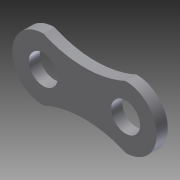
# Autodesk Inventor part: outter_link
Saved by Autodesk Inventor 2011 SP1 (Build 150282100, 282)
## iProperties
Created: 2013-01-14
Part Number: outter_link
Document SubType Name: Modeling
Designer: 971065
Density: 1 g/cm^3
Author: 971065
Autodesk Inventor part; units mm, degrees
ref_plane "YZ Plane" through (0, 0, 0) normal (1, 0, 0) x (0, 1, 0)
ref_plane "XZ Plane" through (0, 0, 0) normal (0, 1, 0) x (-1, 0, 0)
ref_plane "XY Plane" through (0, 0, 0) normal (0, 0, 1) x (1, 0, 0)
sketch "Sketch1" plane through (0, 0, 0) normal (0, 0, 1) x (1, 0, 0)
  arc A0 (-14.097, 3.556) -> (-14.097, -3.556) centre (-14.097, 0) ccw
  arc A1 (-4.699, -3.556) -> (-4.699, 3.556) centre (-4.699, 0) ccw
  line L0 (-9.398, -2.54) -> (-9.398, 2.54)
  arc A2 (-14.097, 3.556) -> (-4.699, 3.556) centre (-9.398, 13.9144) ccw
  arc A3 (-4.699, -3.556) -> (-14.097, -3.556) centre (-9.398, -13.9144) ccw
  circle A4 centre (-14.097, 0) radius 1.651
  circle A5 centre (-4.699, 0) radius 1.651
  point P0 (0, 0)
  dimension "d0" = 7.112
  dimension "d1" = 7.112
  dimension "d5" = 9.398
  dimension "d6" = 4.699
  dimension "d8" = 5.08
  dimension "d9" = 2.54
  dimension "d10" = 4.699
  dimension "d11" = 3.302
  dimension "d12" = 3.302
  constraints: 10 point on circle, 6 centre point, 2 coincident, 2 end point, 1 vertical
  measures "d0" diameter of A0
  measures "d1" diameter of A1
  measures "d5" distance of A1.centre A0.centre
  measures "d6" distance of A1.centre point (0, 0)
  measures "d8" distance of L0.start L0.end
  measures "d9" vertical distance of A1.centre L0.end
  measures "d10" distance from line of L0 A1.centre
  measures "d11" diameter of A5
  measures "d12" diameter of A4
extrude "Extrusion1" add sketch "Sketch1" along normal blind 1.27
body "Solid1"
